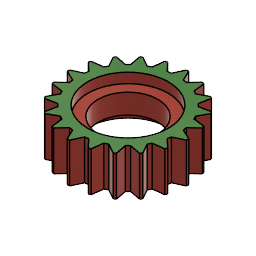
ex29p5 (Autodesk Fusion 360 design; units mm, degrees)
part number: 2026-08-29-11-49-39-336
Autodesk Fusion 360 part; units mm, degrees
sketch "Sketch1" plane through (0, 0, 0) normal (0, 1, 0) x (1, 0, 0)
  circle A0 centre (0, 0) radius 20.25
  circle A1 centre (0, 0) radius 15
  line L0 (-30, 0.6) -> (-30, -0.6)
  line L1 (30, -0.6) -> (30, 0.6)
  line L2 (30, 0.6) -> (24.8219, 2.9786)
  line L3 (24.995, -0.4999) -> (25, -0.5) construction
  line L4 (29.994, -0.5999) -> (30, -0.6) construction
  line L5 (30, 0.6) -> (29.994, 0.5999) construction
  line L6 (25, 0.5) -> (24.995, 0.4999) construction
  line L7 (25, 3) -> (25, 2.8968)
  line L8 (24.8193, -3) -> (30, -0.6)
  line L9 (25, -3) -> (24.8193, -3)
  line L10 (-25, -3) -> (-24.8219, -2.9786) construction
  line L11 (30, 0.6) -> (29.994, 0.6)
  line L12 (24.8193, 3) -> (25, 3)
  line L13 (29.994, -0.6) -> (30, -0.6)
  line L14 (14.8932, 1.7872) -> (20.1058, 2.4127) construction
  line L15 (24.8219, 2.9786) -> (25, 3) construction
  line L16 (28.7171, 8.6999) -> (28.3463, 9.8411)
  line L17 (24.5317, 4.8164) -> (28.7171, 8.6999)
  line L18 (28.3463, 9.8411) -> (22.6866, 10.5032)
  line L19 (24.6232, 17.1481) -> (23.9178, 18.119)
  line L20 (21.8426, 12.1614) -> (24.6232, 17.1481)
  line L21 (23.9178, 18.119) -> (18.3306, 16.9997)
  line L22 (18.119, 23.9178) -> (17.1481, 24.6232)
  line L23 (17.0155, 18.3159) -> (18.119, 23.9178)
  line L24 (17.1481, 24.6232) -> (12.1802, 21.8322)
  line L25 (9.8411, 28.3463) -> (8.6999, 28.7171)
  line L26 (10.5228, 22.6776) -> (9.8411, 28.3463)
  line L27 (8.6999, 28.7171) -> (4.8375, 24.5275)
  line L28 (0.6, 30) -> (-0.6, 30)
  line L29 (3, 24.8193) -> (0.6, 30)
  line L30 (-0.6, 30) -> (-2.9786, 24.8219)
  line L31 (-8.6999, 28.7171) -> (-9.8411, 28.3463)
  line L32 (-4.8164, 24.5317) -> (-8.6999, 28.7171)
  line L33 (-9.8411, 28.3463) -> (-10.5032, 22.6866)
  line L34 (-17.1481, 24.6232) -> (-18.119, 23.9178)
  line L35 (-12.1614, 21.8426) -> (-17.1481, 24.6232)
  line L36 (-18.119, 23.9178) -> (-16.9997, 18.3306)
  line L37 (-23.9178, 18.119) -> (-24.6232, 17.1481)
  line L38 (-18.3159, 17.0155) -> (-23.9178, 18.119)
  line L39 (-24.6232, 17.1481) -> (-21.8322, 12.1802)
  line L40 (-28.3463, 9.8411) -> (-28.7171, 8.6999)
  line L41 (-22.6776, 10.5228) -> (-28.3463, 9.8411)
  line L42 (-28.7171, 8.6999) -> (-24.5275, 4.8375)
  line L43 (-30, 0.6) -> (-30, -0.6)
  line L44 (-24.8193, 3) -> (-30, 0.6)
  line L45 (-30, -0.6) -> (-24.8219, -2.9786)
  line L46 (-28.7171, -8.6999) -> (-28.3463, -9.8411)
  line L47 (-24.5317, -4.8164) -> (-28.7171, -8.6999)
  line L48 (-28.3463, -9.8411) -> (-22.6866, -10.5032)
  line L49 (-24.6232, -17.1481) -> (-23.9178, -18.119)
  line L50 (-21.8426, -12.1614) -> (-24.6232, -17.1481)
  line L51 (-23.9178, -18.119) -> (-18.3306, -16.9997)
  line L52 (-18.119, -23.9178) -> (-17.1481, -24.6232)
  line L53 (-17.0155, -18.3159) -> (-18.119, -23.9178)
  line L54 (-17.1481, -24.6232) -> (-12.1802, -21.8322)
  line L55 (-9.8411, -28.3463) -> (-8.6999, -28.7171)
  line L56 (-10.5228, -22.6776) -> (-9.8411, -28.3463)
  line L57 (-8.6999, -28.7171) -> (-4.8375, -24.5275)
  line L58 (-0.6, -30) -> (0.6, -30)
  line L59 (-3, -24.8193) -> (-0.6, -30)
  line L60 (0.6, -30) -> (2.9786, -24.8219)
  line L61 (8.6999, -28.7171) -> (9.8411, -28.3463)
  line L62 (4.8164, -24.5317) -> (8.6999, -28.7171)
  line L63 (9.8411, -28.3463) -> (10.5032, -22.6866)
  line L64 (17.1481, -24.6232) -> (18.119, -23.9178)
  line L65 (12.1614, -21.8426) -> (17.1481, -24.6232)
  line L66 (18.119, -23.9178) -> (16.9997, -18.3306)
  line L67 (23.9178, -18.119) -> (24.6232, -17.1481)
  line L68 (18.3159, -17.0155) -> (23.9178, -18.119)
  line L69 (24.6232, -17.1481) -> (21.8322, -12.1802)
  line L70 (28.3463, -9.8411) -> (28.7171, -8.6999)
  line L71 (22.6776, -10.5228) -> (28.3463, -9.8411)
  line L72 (28.7171, -8.6999) -> (24.5275, -4.8375)
  arc A2 (12.1802, 21.8322) -> (10.5228, 22.6776) centre (0, 0) ccw
  arc A3 (4.8375, 24.5275) -> (3, 24.8193) centre (0, 0) ccw
  arc A4 (-2.9786, 24.8219) -> (-4.8164, 24.5317) centre (0, 0) ccw
  arc A5 (-10.5032, 22.6866) -> (-12.1614, 21.8426) centre (0, 0) ccw
  arc A6 (-16.9997, 18.3306) -> (-18.3159, 17.0155) centre (0, 0) ccw
  arc A7 (-21.8322, 12.1802) -> (-22.6776, 10.5228) centre (0, 0) ccw
  line L73 (-24.8193, -3) -> (-25, -3)
  line L74 (-24.8219, 2.9786) -> (-25, 3) construction
  line L75 (-25, 3) -> (-24.8193, 3)
  line L76 (-24.9928, 0.6) -> (-25, 0.6)
  line L77 (-25, 0.5) -> (-24.995, 0.4999) construction
  line L78 (-25, -0.6) -> (-24.9928, -0.6)
  line L79 (-24.995, -0.4999) -> (-25, -0.5) construction
  arc A8 (-24.5275, 4.8375) -> (-24.8219, 2.9786) centre (0, 0) ccw
  line L80 (-25, 2.9163) -> (-25, 3)
  line L81 (-25, -3) -> (-25, -2.8968)
  arc A9 (-24.8219, -2.9786) -> (-24.5317, -4.8164) centre (0, 0) ccw
  arc A10 (-22.6866, -10.5032) -> (-21.8426, -12.1614) centre (0, 0) ccw
  arc A11 (-18.3306, -16.9997) -> (-17.0155, -18.3159) centre (0, 0) ccw
  arc A12 (-12.1802, -21.8322) -> (-10.5228, -22.6776) centre (0, 0) ccw
  arc A13 (-4.8375, -24.5275) -> (-3, -24.8193) centre (0, 0) ccw
  arc A14 (2.9786, -24.8219) -> (4.8164, -24.5317) centre (0, 0) ccw
  arc A15 (10.5032, -22.6866) -> (12.1614, -21.8426) centre (0, 0) ccw
  arc A16 (24.5275, -4.8375) -> (24.8193, -3) centre (0, 0) ccw
  arc A17 (24.8219, 2.9786) -> (24.5317, 4.8164) centre (0, 0) ccw
  arc A18 (22.6866, 10.5032) -> (21.8426, 12.1614) centre (0, 0) ccw
  arc A19 (18.3306, 16.9997) -> (17.0155, 18.3159) centre (0, 0) ccw
  arc A20 (16.9997, -18.3306) -> (18.3159, -17.0155) centre (0, 0) ccw
  arc A21 (21.8322, -12.1802) -> (22.6776, -10.5228) centre (0, 0) ccw
  dimension "d2" = 40.5
  dimension "d3" = 30
  dimension "d4" = 50
  dimension "d5" = 50
  dimension "d6" = 6
  dimension "d7" = 60
  dimension "d8" = 1.2
  dimension "d10" = 360
  constraint coincident A0.centre A1.centre
  constraint concentric A1 A17
  constraint horizontal L9
  constraint perpendicular L73 L81
  constraint parallel L9 L12
  constraint parallel L7 L80
  constraint coincident A0.centre L14
  constraint horizontal L11
  constraint perpendicular L0 L76
  constraint parallel L0 L1
  constraint collinear L3 L4
  constraint collinear L5 L6
  constraint coincident L2 L7.end
  constraint collinear L10 L14
  constraint coincident A1 L14.start
  constraint coincident A0 L14.end
  constraint collinear L14 L15
  constraint coincident L12.start A17
  constraint concentric A2 A19
  constraint concentric A2 A3
  constraint concentric A3 A4
  constraint concentric A4 A5
  constraint concentric A5 A6
  constraint concentric A6 A7
  constraint concentric A7 A8
  constraint coincident L73.start A9
  constraint coincident L44 L80.start
  constraint coincident L45 L81.end
  constraint concentric A9 A10
  constraint concentric A10 A11
  constraint concentric A11 A12
  constraint concentric A12 A13
  constraint concentric A13 A14
  constraint concentric A14 A15
  constraint concentric A15 A20
  constraint concentric A16 A21
  constraint concentric A17 A18
  constraint concentric A18 A19
  constraint concentric A20 A21
  measures "d2" diameter of A0
  measures "d3" diameter of A1
  measures "d4" diameter of A17
  measures "d5" distance of L74.end L7.start
  measures "d6" distance of L10.start L74.end
  measures "d7" distance of L0.end L1.start
  measures "d8" distance of L0.start L0.end
extrude "Extrude1" add sketch "Sketch1" along normal blind 20 contours L0 L1 L2 L8 L16 L17 L18 L19 L20 L21 L22 L23 L24 L25 L26 L27 L28 L29 L30 L31 L32 L33 L34 L35 L36 L37 L38 L39 L40 L41 L42 L43 L44 L45 L46 L47 L48 L49 L50 L51 L52 L53 L54 L55 L56 L57 L58 L59 L60 L61 L62 L63 L64 L65 L66 L67 L68 L69 L70 L71 L72 A2 A3 A4 A5 A6 A7 A8 A9 A10 A11 A12 A13 A14 A15 A16 A17 A18 A19 A20 A21
extrude "Extrude2" add sketch "Sketch1" along normal blind 10 from surface at 5 contours A0
